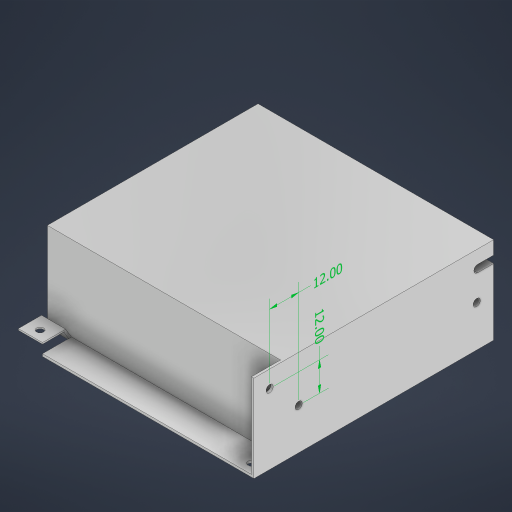
# Autodesk Inventor part: smps
Saved by Autodesk Inventor 2024 (Build 280153000, 153)
## iProperties
Created: 2023-07-11
Part Number: smps
Material: 일반
Document SubType Name: Modeling
Designer: 6gioc
Density: 1 g/cm^3
Appearance: 기본값
Author: 6gioc
Autodesk Inventor part; units mm, degrees
ref_plane "YZ Plane" through (0, 0, 0) normal (1, 0, 0) x (0, 1, 0)
ref_plane "XZ Plane" through (0, 0, 0) normal (0, 1, 0) x (-1, 0, 0)
ref_plane "XY Plane" through (0, 0, 0) normal (0, 0, 1) x (1, 0, 0)
sketch "스케치1" plane through (0, 0, 0) normal (0, 1, 0) x (-1, 0, 0)
  line L0 (0, 0) -> (97.5, 0)
  line L1 (97.5, 0) -> (97.5, -99.2)
  line L2 (97.5, -99.2) -> (0, -99.2)
  line L3 (0, -99.2) -> (0, 0)
  line L4 (97.5, 0) -> (1, 0)
  line L5 (1, 0) -> (1, -12)
  line L6 (1, -12) -> (97.5, -12)
  line L7 (97.5, -12) -> (97.5, 0)
  point P0 (1, -6)
  point P1 (97.5, -6)
  point P2 (48.75, 0)
  dimension "d0" = 97.5
  dimension "d1" = 99.2
  dimension "d2" = 96.5
  dimension "d3" = 12
  dimension "d6" = 1
  constraints: 16 end point, 4 parallel, 3 midpoint, 2 horizontal, 2 perpendicular, 1 point on line
  measures "d0" distance of L1.end L2.end
  measures "d1" distance of L0.end L1.end
  measures "d2" distance of L6.end L5.end
  measures "d3" distance of L5.end L4.end
  measures "d6" distance between parallel lines of L5 L3
sketch "스케치1 outline for 돌출1" plane through (0, 0, 0) normal (0, 1, 0) x (-1, 0, 0)
  line L0 (0, 0) -> (0, -99.2)
  line L1 (1, 0) -> (0, 0)
  line L2 (1, -12) -> (1, 0)
  line L3 (97.5, -12) -> (1, -12)
  line L4 (97.5, -99.2) -> (97.5, -12)
  line L5 (0, -99.2) -> (97.5, -99.2)
extrude "돌출1" add sketch "스케치1 outline for 돌출1" along normal blind 36
sketch "스케치1 outline for 돌출2" plane through (0, 0, 0) normal (0, 1, 0) x (-1, 0, 0)
  line L0 (1, -12) -> (97.5, -12)
  line L1 (1, 0) -> (1, -12)
  line L2 (97.5, 0) -> (1, 0)
  line L3 (97.5, -12) -> (97.5, 0)
extrude "돌출2" add sketch "스케치1 outline for 돌출2" along normal blind 1
sketch "스케치2" plane through (0, 1, 0) normal (0, 1, 0) x (1, 0, 0)
  circle A0 centre (-5, 4) radius 1.5
  line L0 (0, 0) -> (0, 99.2) projected
  line L1 (-97.5, 0) -> (-1, 0) projected
  line L2 (-97.5, 0) -> (0, 0) projected
  line L3 (-97.5, 0) -> (-87.5, 0)
  line L4 (-87.5, 0) -> (-87.5, 9)
  line L5 (-87.5, 9) -> (-97.5, 9)
  line L6 (-97.5, 9) -> (-97.5, 0)
  dimension "d11" = 3
  dimension "d13" = 5
  dimension "d14" = 4
  dimension "d15" = 10
  dimension "d16" = 9
  constraints: 8 end point, 2 parallel, 1 centre point, 1 horizontal, 1 perpendicular
  measures "d11" diameter of A0
  measures "d13" distance from line of L0 A0.centre
  measures "d14" distance from line of L1 A0.centre
  measures "d15" distance of L5.end L4.end
  measures "d16" distance of L4.end L3.end
sketch "스케치2 outline for 돌출3" plane through (0, 1, 0) normal (0, 1, 0) x (1, 0, 0)
  line L0 (-97.5, 9) -> (-97.5, 0)
  line L1 (-87.5, 9) -> (-97.5, 9)
  line L2 (-87.5, 0) -> (-87.5, 9)
  line L3 (-97.5, 0) -> (-87.5, 0)
extrude "돌출3" cut sketch "스케치2 outline for 돌출3" against normal blind 1
sketch "스케치2 outline for 돌출4" plane through (0, 1, 0) normal (0, 1, 0) x (1, 0, 0)
  line L0 (-97.5, 9) -> (-97.5, 0)
  line L1 (-87.5, 9) -> (-97.5, 9)
  line L2 (-87.5, 0) -> (-87.5, 9)
  line L3 (-97.5, 0) -> (-87.5, 0)
extrude "돌출4" add sketch "스케치2 outline for 돌출4" along normal blind 4
sketch "스케치2 outline for 돌출5" plane through (0, 1, 0) normal (0, 1, 0) x (1, 0, 0)
  line L0 (-97.5, 9) -> (-97.5, 0)
  line L1 (-87.5, 9) -> (-97.5, 9)
  line L2 (-87.5, 0) -> (-87.5, 9)
  line L3 (-97.5, 0) -> (-87.5, 0)
extrude "돌출5" cut sketch "스케치2 outline for 돌출5" along normal blind 3.4
sketch "스케치3" plane through (-87.5, 5, -9) normal (0, 0, -1) x (-1, 0, 0)
  line L0 (0, 0) -> (10, 0)
  line L1 (10, 0) -> (10, -4)
  line L2 (10, -4) -> (0, -4)
  line L3 (0, -4) -> (0, 0)
  point P0 (-87.5, -5)
  point P1 (0, -0.6)
  constraints: 8 end point, 2 parallel, 1 horizontal, 1 perpendicular, 1 point on line
sketch "스케치3 outline for 돌출6" plane through (-87.5, 5, -9) normal (0, 0, -1) x (-1, 0, 0)
  line L0 (0, 0) -> (0, -4)
  line L1 (10, 0) -> (0, 0)
  line L2 (10, -4) -> (10, 0)
  line L3 (0, -4) -> (10, -4)
extrude "돌출6" add sketch "스케치3 outline for 돌출6" along normal blind 0.6
chamfer "모따기1" distance 2.4 distance2 4 1 edges at (-92.5, 1, -9.6) measured on face at (-29.8333, 1, -7)
chamfer "모따기2" distance 2.4 distance2 4 1 edges at (-92.5, 0, -9)
sketch "스케치4" plane through (0, 5, 0) normal (0, 1, 0) x (1, 0, 0)
  circle A0 centre (-92.5, 4) radius 1.5
  line L0 (-97.5, 0) -> (-97.5, 9.6) projected
  line L1 (-97.5, 0) -> (-87.5, 0) projected
  point P0 (0, 0)
  point P1 (-97.5, 4.8)
  dimension "d31" = 3
  dimension "d32" = 5
  dimension "d33" = 4
  constraints: 1 centre point, 1 midpoint
  measures "d31" diameter of A0
  measures "d32" horizontal distance of point (-97.5, 4.8) A0.centre
  measures "d33" distance from line of L1 A0.centre
sketch "스케치2 outline for 돌출7" plane through (0, 1, 0) normal (0, 1, 0) x (1, 0, 0)
  circle A0 centre (-5, 4) radius 1.5
extrude "돌출7" cut sketch "스케치2 outline for 돌출7" against normal blind 3.1
sketch "스케치4 outline for 돌출8" plane through (0, 5, 0) normal (0, 1, 0) x (1, 0, 0)
  circle A0 centre (-92.5, 4) radius 1.5
extrude "돌출8" cut sketch "스케치4 outline for 돌출8" against normal blind 3.1
sketch "스케치5" plane through (0, 0, 0) normal (1, 0, 0) x (0, 0, -1)
  circle A0 centre (18.5, 17) radius 1.5
  circle A1 centre (92.2, 17) radius 1.5
  line L0 (0, 0) -> (99.2, 0) projected
  line L1 (99.2, 0) -> (99.2, 36) projected
  circle A2 centre (6.5, 29) radius 1.5
  circle A3 centre (92.5, 29) radius 1.5
  line L2 (0, 36) -> (99.2, 36) projected
  line L3 (0, 0) -> (0, 36) projected
  line L4 (92.5, 30.5) -> (99.2, 30.5)
  line L5 (99.2, 30.5) -> (99.2, 27.5)
  line L6 (99.2, 27.5) -> (92.5, 27.5)
  line L7 (92.5, 27.5) -> (92.5, 30.5)
  dimension "d44" = 3
  dimension "d38" = 3
  dimension "d39" = 3
  dimension "d40" = 17
  dimension "d41" = 73.7
  dimension "d42" = 7
  dimension "d43" = 3
  dimension "d45" = 7
  dimension "d46" = 6.5
  dimension "d48" = 86
  constraints: 8 end point, 3 centre point, 2 horizontal alignment, 2 parallel, 1 horizontal, 1 perpendicular, 1 point on line, 3 other
  measures "d38" diameter of A0
  measures "d39" diameter of A1
  measures "d40" distance from line of L0 A1.centre
  measures "d41" distance of A1.centre A0.centre
  measures "d42" distance from line of L1 A1.centre
  measures "d43" diameter of A2
  measures "d45" distance from line of L2 A2.centre
  measures "d46" distance from line of L3 A2.centre
  measures "d48" distance of point (92.5, 29) A2.centre
sketch "스케치5 outline for 돌출9" plane through (0, 0, 0) normal (1, 0, 0) x (0, 0, -1)
  circle A0 centre (6.5, 29) radius 1.5
  circle A1 centre (18.5, 17) radius 1.5
  line L0 (92.5, 27.5) -> (99.2, 27.5)
  arc A2 (92.5, 30.5) -> (92.5, 27.5) centre (92.5, 29) ccw
  line L1 (99.2, 30.5) -> (92.5, 30.5)
  line L2 (99.2, 27.5) -> (99.2, 30.5)
  circle A3 centre (92.2, 17) radius 1.5
extrude "돌출9" cut sketch "스케치5 outline for 돌출9" against normal blind 3
